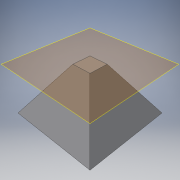
# Autodesk Inventor part: hologram pyramid (for assembly)
Saved by Autodesk Inventor 2016 (Build 200138000, 138)
## iProperties
Created: 2017-10-23
Part Number: hologram pyramid (for assembly)
Material: Generic
Document SubType Name: Modeling
Designer: student
Density: 1 g/cm^3
Appearance: Default
Author: student
Autodesk Inventor part; units mm, degrees
ref_plane "YZ Plane" through (0, 0, 0) normal (1, 0, 0) x (0, 1, 0)
ref_plane "XY Plane" through (0, 0, 0) normal (0, 0, 1) x (1, 0, 0)
sketch "Sketch1" plane through (0, 0, 0) normal (0, 1, 0) x (-1, 0, 0)
  line L0 (-149.225, 149.225) -> (149.225, 149.225)
  line L1 (149.225, 149.225) -> (149.225, -149.225)
  line L2 (149.225, -149.225) -> (-149.225, -149.225)
  line L3 (-149.225, -149.225) -> (-149.225, 149.225)
  line L4 (-149.225, 149.225) -> (149.225, -149.225) construction
  line L5 (149.225, 149.225) -> (-149.225, -149.225) construction
  point P0 (0, 0)
  dimension "d0" = 298.45
  dimension "d1" = 298.45
  constraints: 12 end point, 2 midpoint, 2 parallel, 1 horizontal, 1 perpendicular
  measures "d0" distance of L0.end L1.end
  measures "d1" distance of L1.end L2.end
ref_plane "Work Plane1" through (0, 165.1, 0) normal (0, 1, 0) x (-1, 0, 0)
sketch "Sketch2" plane through (0, 165.1, 0) normal (0, 1, 0) x (-1, 0, 0)
  line L0 (-31.75, 31.75) -> (31.75, 31.75)
  line L1 (31.75, 31.75) -> (31.75, -31.75)
  line L2 (31.75, -31.75) -> (-31.75, -31.75)
  line L3 (-31.75, -31.75) -> (-31.75, 31.75)
  line L4 (-31.75, 31.75) -> (31.75, -31.75) construction
  line L5 (31.75, 31.75) -> (-31.75, -31.75) construction
  point P0 (0, 0)
  dimension "d3" = 63.5
  dimension "d4" = 63.5
  constraints: 12 end point, 2 midpoint, 2 parallel, 1 horizontal, 1 perpendicular
  measures "d3" distance of L1.end L2.end
  measures "d4" distance of L0.end L1.end
loft "Loft1" add profiles "Sketch2", "Sketch1"
shell "Shell1" thickness 2.54 removed faces 1 at (-49.7417, 0, -49.7417)
body "Solid1"
